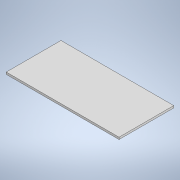
# Autodesk Inventor part: Etage
Saved by Autodesk Inventor 2020 (Build 240168000, 168)
## iProperties
Created: 2019-11-28
Part Number: Etage
Material: Générique
Document SubType Name: Modeling
Designer: erwan
Density: 1 g/cm^3
Appearance: Par défaut
Author: erwan
Autodesk Inventor part; units mm, degrees
ref_plane "YZ Plane" through (0, 0, 0) normal (1, 0, 0) x (0, 1, 0)
ref_plane "XZ Plane" through (0, 0, 0) normal (0, 1, 0) x (-1, 0, 0)
ref_plane "XY Plane" through (0, 0, 0) normal (0, 0, 1) x (1, 0, 0)
sketch "Esquisse1" plane through (0, 0, 0) normal (0, 1, 0) x (-1, 0, 0)
  line L0 (-165, 80) -> (165, 80)
  line L1 (165, 80) -> (165, -80)
  line L2 (165, -80) -> (-165, -80)
  line L3 (-165, -80) -> (-165, 80)
  line L4 (-165, 80) -> (165, -80) construction
  line L5 (165, 80) -> (-165, -80) construction
  point P0 (0, 0)
  dimension "d0" = 330
  dimension "d1" = 160
  constraints: 12 end point, 2 midpoint, 2 parallel, 1 horizontal, 1 perpendicular
  measures "d0" distance of L1.end L2.end
  measures "d1" distance of L0.end L1.end
extrude "Extrusion1" add sketch "Esquisse1" along normal blind 6
